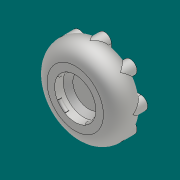
# Autodesk Inventor part: finger2
Saved by Autodesk Inventor 2018.2 (Build 222227000, 227)
## iProperties
Created: 2020-12-02
Part Number: finger2
Material: アルミニウム 6061
Document SubType Name: Modeling
Designer: gisen
Density: 2.7 g/cm^3
Appearance: アルミニウム - フラット
Author: gisen
Autodesk Inventor part; units mm, degrees
ref_plane "YZ Plane" through (0, 0, 0) normal (1, 0, 0) x (0, 1, 0)
ref_plane "XZ Plane" through (0, 0, 0) normal (0, 1, 0) x (-1, 0, 0)
ref_plane "XY Plane" through (0, 0, 0) normal (0, 0, 1) x (1, 0, 0)
sketch "スケッチ1" plane through (0, 0, 0) normal (0, 0, 1) x (1, 0, 0)
  line L0 (0, 0) -> (3.85, 0) construction
  line L1 (3.85, 0) -> (3.85, 1.7) construction
  line L2 (3.85, 1.7) -> (0, 1.7) construction
  line L3 (0, 1.7) -> (0, 0) construction
  line L4 (2.95, 1.7) -> (3.85, 0.8) construction
  line L5 (0, 4.7) -> (5.25, 4.7) construction
  arc A0 (5.25, -0.8) -> (5.25, 4.7) centre (5.25, 1.95) ccw
  line L6 (5.25, 4.7) -> (5.25, -0.8) construction
  arc A1 (3.85, 0) -> (3.85, -0.8) centre (3.9667, -0.4) ccw
  line L7 (3.85, -0.8) -> (5.25, -0.8)
  line L8 (3.9667, -0.4) -> (3.55, -0.4) construction
  line L9 (5.25, 1.95) -> (8, 1.95) construction
  line L10 (0, 4.7) -> (0, 1.7) construction
  line L11 (0, 1.7) -> (2.95, 1.7)
  line L12 (2.95, 1.7) -> (3.85, 0.8)
  line L13 (3.85, 0.8) -> (3.85, 0)
  line L14 (0, 1.7) -> (0, 3.2)
  line L15 (5.25, 4.7) -> (4.25, 4.7)
  arc A2 (0, 3.2) -> (4.25, 4.7) centre (0, 9.9708) ccw
  point P0 (3.7583, -0.4)
  dimension "d0" = 1.7
  dimension "d1" = 3.85
  dimension "d2" = 45
  dimension "d3" = 0.8
  dimension "d4" = 3
  dimension "d5" = 5.5
  dimension "d6" = 0.8
  dimension "d7" = 0.4
  dimension "d8" = 0.3
  dimension "d9" = 8
  dimension "d25" = 1
  dimension "d26" = 1.5
  constraints: 32 end point, 9 point on circle, 5 point on line, 4 horizontal, 3 centre point, 3 midpoint, 2 parallel, 1 horizontal alignment, 1 perpendicular, 1 tangent
  measures "d0" distance between parallel lines of L0 L2
  measures "d1" distance between parallel lines of L3 L1
  measures "d2" angle of L4 L2
  measures "d3" distance of L0.end L4.end
  measures "d4" distance between parallel lines of L2 L5
  measures "d5" distance of L5.end L6.end
  measures "d6" distance from line of L6.end L0
  measures "d7" distance from line of L7 L8.start
  measures "d8" distance from line of L1 L8.end
  measures "d9" distance from line of L3 L9.end
  measures "d25" distance from line of L6 L15.end
  measures "d26" distance from line of L5 L14.end
revolve "回転1" add sketch "スケッチ1" angle 360 about axis through (0, 4.7, 0) along (0, -1, 0)
sketch "スケッチ2" plane through (0, -0.8, 0) normal (0, -1, 0) x (1, 0, 0)
  circle A0 centre (0, 0) radius 3.85 construction
  line L0 (0, 0) -> (1.925, -3.3342)
  line L1 (0, 0) -> (-1.925, -3.3342)
  arc A1 (-1.925, -3.3342) -> (1.925, -3.3342) centre (0, 0) ccw
  line L2 (0, 0) -> (0, -3.85) construction
  line L3 (0, 0) -> (3.3342, 1.925)
  line L4 (0, 0) -> (3.3342, -1.925)
  arc A2 (3.3342, -1.925) -> (3.3342, 1.925) centre (0, 0) ccw
  line L5 (0, 0) -> (3.85, 0) construction
  line L6 (0, 0) -> (-1.925, 3.3342)
  line L7 (0, 0) -> (1.925, 3.3342)
  arc A3 (1.925, 3.3342) -> (-1.925, 3.3342) centre (0, 0) ccw
  line L8 (0, 0) -> (0, 3.85) construction
  line L9 (0, 0) -> (-3.3342, -1.925)
  line L10 (0, 0) -> (-3.3342, 1.925)
  arc A4 (-3.3342, 1.925) -> (-3.3342, -1.925) centre (0, 0) ccw
  line L11 (0, 0) -> (-3.85, 0) construction
  point P0 (0, 0)
  point P1 (0, 0)
  point P2 (0, 0)
  dimension "d11" = 60
  dimension "d12" = 30
  dimension "d15" = 360
  constraints: 24 end point, 14 point on circle, 6 coincident, 4 centre point, 1 vertical, 39 other
  measures "d11" angle of L1 L0
  measures "d12" angle of L2 L0
extrude "押し出し1" cut sketch "スケッチ2" against normal blind 0.8
sketch "スケッチ3" plane through (0, 4.7, 0) normal (0, 1, 0) x (1, 0, 0)
  line L0 (-4.8163, 0) -> (-6.75, 0) construction
  line L1 (-4.8163, 1.25) -> (-6.75, 1.25)
  line L2 (-6.75, -1.25) -> (-4.8163, -1.25)
  arc A0 (-6.75, 1.25) -> (-6.75, -1.25) centre (-6.75, 0) ccw
  circle A1 centre (0, 0) radius 8 construction
  arc A2 (-4.8163, 1.25) -> (-4.8163, -1.25) centre (0, 0) ccw
  point P0 (-5.7831, 0)
  dimension "d19" = 1.25
  constraints: 8 end point, 4 point on circle, 3 tangent, 2 centre point, 1 coincident, 1 horizontal, 1 midpoint, 1 parallel, 1 point on line
  measures "d19" radius of A0
extrude "押し出し2" add sketch "スケッチ3" against normal blind 2.75
pattern_circular "円形状パターン1" count 8 over 360 about axis through (0, 0.4, 0) along (0, -1, 0) of "押し出し2"
equation "\"d7\" = 0.5 * d6"
equation "\"d12\" = 0.5 * d11"
